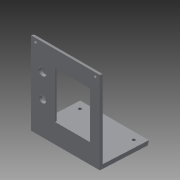
# Autodesk Inventor part: Dekel
Saved by Autodesk Inventor 2015 SP2 (Build 190223200, 223)
## iProperties
Created: 2018-06-26
Part Number: Dekel
Material: Generisch
Document SubType Name: Modeling
Designer: loetscher_l
Density: 1 g/cm^3
Appearance: Vorgabe
Author: loetscher_l
Autodesk Inventor part; units mm, degrees
ref_plane "YZ Plane" through (0, 0, 0) normal (1, 0, 0) x (0, 1, 0)
ref_plane "XZ Plane" through (0, 0, 0) normal (0, 1, 0) x (-1, 0, 0)
ref_plane "XY Plane" through (0, 0, 0) normal (0, 0, 1) x (1, 0, 0)
sketch "Skizze1" plane through (0, 0, 0) normal (0, 1, 0) x (-1, 0, 0)
  line L0 (0, 0) -> (69, 0)
  line L1 (69, 0) -> (69, -78.309)
  line L2 (69, -78.309) -> (0, -78.309)
  line L3 (0, -78.309) -> (0, 0)
  dimension "d0" = 69
  dimension "d1" = 78.309
  constraints: 8 end point, 2 parallel, 1 horizontal, 1 perpendicular
  measures "d0" distance of L1.end L2.end
  measures "d1" distance of L0.end L1.end
extrude "Extrusion1" add sketch "Skizze1" against normal blind 3
ref_plane "Arbeitsebene1" through (-69, 0, -78.309) normal (0, -0.0498957, -0.9987544) x (1, 0, 0)
sketch "Skizze2" plane through (-69, 0, -78.309) normal (0, -0.0498957, -0.9987544) x (1, 0, 0)
  line L0 (0, 0) -> (69, 0) projected
  line L1 (69, 0) -> (69, 2.9963) projected
  line L2 (0, 2.9963) -> (69, 2.9963) projected
  line L3 (0, 0) -> (0, 2.9963) projected
  line L4 (69, 0) -> (0, 0)
  line L5 (0, 0) -> (0, -46.352)
  line L6 (0, -46.352) -> (69, -46.352)
  line L7 (69, -46.352) -> (69, 0)
  point P0 (69, 3.9073)
  dimension "d5" = 69
  dimension "d6" = 46.352
  constraints: 8 end point, 2 parallel, 1 horizontal, 1 perpendicular
  measures "d5" distance of L6.end L5.end
  measures "d6" distance of L5.end L4.end
extrude "Extrusion2" add sketch "Skizze2" along normal blind 4 contours L0 L7 L6 L5
sketch "Skizze4" plane through (-69, 0, -78.309) normal (0, 0.0498957, 0.9987544) x (1, 0, 0)
  line L0 (0, 0) -> (0, 46.352) projected
  line L1 (0, 46.352) -> (69, 46.352) projected
  line L2 (69, 46.352) -> (69, 0) projected
  line L3 (0, 0) -> (69, 0) projected
  line L4 (69, 46.352) -> (69, 0) projected
  line L5 (0, 46.352) -> (69, 46.352) projected
  line L6 (0, 0) -> (0, 46.352) projected
  line L7 (69, 0) -> (0, 0) projected
  point P0 (69, -3.9073)
  point P1 (61.5, 38.718)
  point P2 (7.5, 38.718)
  dimension "d12" = 7.634
  dimension "d14" = 7.5
  dimension "d15" = 7.634
  dimension "d16" = 7.5
  measures "d12" distance from line of L1 point (61.5, 38.718)
  measures "d14" distance from line of L2 point (61.5, 38.718)
  measures "d15" distance from line of L1 point (7.5, 38.718)
  measures "d16" distance from line of L0 point (7.5, 38.718)
hole "Bohrung1" at (-7.5, 38.6698, -80.2409) at (-61.5, 38.6698, -80.2409) direction (0, -0.0498957, -0.9987544) diameter 3 depth 8 tip angle 118
sketch "Skizze5" plane through (0, 0, 0) normal (0, 1, 0) x (1, 0, 0)
  line L0 (0, 0) -> (-69, 0) projected
  line L1 (0, 78.309) -> (0, 0) projected
  line L2 (-69, 78.309) -> (0, 78.309) projected
  line L3 (-69, 0) -> (-69, 78.309) projected
  line L4 (-10, 62.55) -> (-44.9, 62.55)
  line L5 (-44.9, 62.55) -> (-44.9, 15.75)
  line L6 (-44.9, 15.75) -> (-10, 15.75)
  line L7 (-10, 15.75) -> (-10, 62.55)
  line L8 (-5, 65.9) -> (-50, 65.9)
  line L9 (-50, 65.9) -> (-50, 12.4)
  line L10 (-50, 12.4) -> (-5, 12.4)
  line L11 (-5, 12.4) -> (-5, 65.9)
  circle A0 centre (-57.5, 25) radius 4
  circle A1 centre (-57.5, 49.009) radius 3.5
  point P0 (-5, 2.588)
  point P1 (-65, 2.588)
  dimension "d24" = 34.9
  dimension "d25" = 46.8
  dimension "d26" = 53.5
  dimension "d27" = 45
  dimension "d28" = 5
  dimension "d29" = 3.35
  dimension "d30" = 12.4
  dimension "d31" = 5
  dimension "d32" = 7
  dimension "d34" = 11.5
  dimension "d35" = 8
  dimension "d37" = 11.5
  dimension "d40" = 5
  dimension "d41" = 2.588
  dimension "d42" = 4
  dimension "d56" = 29.3
  dimension "d57" = 25
  constraints: 16 end point, 4 parallel, 2 centre point, 2 horizontal, 2 perpendicular, 1 horizontal alignment
  measures "d24" distance between parallel lines of L5 L7
  measures "d25" distance between parallel lines of L6 L4
  measures "d26" distance between parallel lines of L10 L8
  measures "d27" distance between parallel lines of L9 L11
  measures "d28" distance between parallel lines of L7 L11
  measures "d29" distance between parallel lines of L10 L6
  measures "d30" distance between parallel lines of L0 L10
  measures "d31" distance between parallel lines of L1 L11
  measures "d32" diameter of A1
  measures "d34" distance from line of L3 A1.centre
  measures "d35" diameter of A0
  measures "d37" distance from line of L3 A0.centre
  measures "d40" distance from line of L1 point (-5, 2.588)
  measures "d41" distance from line of L0 point (-5, 2.588)
  measures "d42" distance from line of L3 point (-65, 2.588)
  measures "d56" distance from line of L2 A1.centre
  measures "d57" distance from line of L0 A0.centre
extrude "Extrusion4" cut sketch "Skizze5" against normal blind 69 contours L7 L6 L5 L4 | A0 | A1
extrude "Extrusion5" cut sketch "Skizze5" against normal blind 1.5 contours L11 L10 L9 L8
hole "Bohrung2" at (-5, 0, -2.588) at (-65, 0, -2.588) direction (0, -1, 0) diameter 3 depth 8 tip angle 118
sketch "Skizze6" plane through (0, 0, -78.309) normal (1, 0, 0) x (0, -0.0498957, -0.9987544)
  line L0 (0, 0) -> (0.1497, -2.9963) projected
  line L1 (0, 0) -> (-78.2115, -3.9073) projected
  line L2 (-78.2115, -3.9073) -> (-78.0618, -6.9035) projected
  line L3 (0.1497, -2.9963) -> (-78.0618, -6.9035) projected
  line L4 (0, 0) -> (0.1497, -2.9963) projected
  line L5 (0, 46.352) -> (0, 0) projected
  line L6 (0, 0) -> (4, 0) projected
  line L7 (4, 46.352) -> (4, 0) projected
  line L8 (0, 46.352) -> (4, 46.352) projected
  line L9 (4, 0) -> (0, 0)
  line L10 (0, 0) -> (4, 0) projected
  line L11 (0, 0) -> (0.1497, -2.9963)
  line L12 (0.1497, -2.9963) -> (4, -2.8039)
  line L13 (4, -2.8039) -> (4, 0)
  line L14 (0.1497, -2.9963) -> (-78.0618, -6.9035) projected
  constraints: 8 end point, 4 coincident, 3 collinear, 2 perpendicular
extrude "Extrusion6" add sketch "Skizze6" against normal blind 69 contours L6 L13 L12 L0
sketch "Skizze7" plane through (-69, -3, 0) normal (-1, 0, 0) x (0, 0, 1)
  line L0 (0, 3) -> (-78.309, 3) projected
  line L1 (-78.309, 3) -> (-80.6218, 49.2943) projected
  line L2 (-80.6218, 49.2943) -> (-84.6168, 49.0947) projected
  line L3 (-84.6168, 49.0947) -> (-82.1641, 0) projected
  line L4 (0, 0) -> (-82.1641, 0) projected
  line L5 (0, 3) -> (0, 0) projected
  line L6 (-78.309, 3) -> (-80.6218, 49.2943) projected
  line L7 (-84.6168, 49.0947) -> (-82.1641, 0) projected
  line L8 (-84.5633, 48.0242) -> (-80.6218, 49.2943)
  line L9 (0, 0) -> (0, 3)
  line L10 (0, 0) -> (0, 3)
  line L11 (0, 3) -> (0.8038, 0)
  line L12 (0.8038, 0) -> (0, 0)
  line L13 (0.8038, 0) -> (0, 0)
  line L14 (0, 0) -> (0, 3)
  line L15 (0, 3) -> (0.8038, 3)
  line L16 (0.8038, 3) -> (0.8038, 0)
  line L17 (0, 0) -> (0, 3)
  line L18 (0, 3) -> (0, 0) projected
  point P0 (-0.4568, 4.2362)
  dimension "d59" = 15
  dimension "d62" = 15
  constraints: 20 end point, 4 equal length, 3 coincident, 3 perpendicular, 1 horizontal, 1 point on line
  measures "d59" angle of L8 L2
  measures "d62" angle of L11 L5
extrude "Extrusion7" cut sketch "Skizze7" against normal blind 80 contours L8 L3 L2
extrude "Extrusion8" add sketch "Skizze7" against normal blind 69 contours L11 L12 L5
